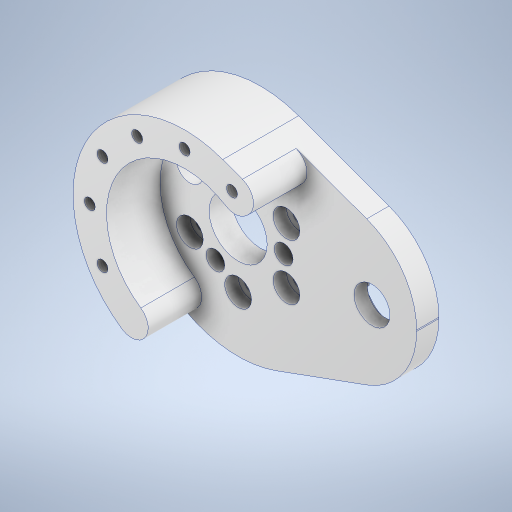
# Autodesk Inventor part: RP_Thigh-Base
Saved by Autodesk Inventor 2024.3 (Build 283343000, 343)
## iProperties
Created: 2024-10-20
Part Number: RP_Thigh-Base
Material: アルミニウム 6061
Document SubType Name: Sheet Metal
Designer: 佐藤智貴
Density: 2.7 g/cm^3
Appearance: アルミニウム - フラット
Mass: 44.9931 g
Surface Area: 86.4883 cm^2
Volume: 16.6641 cm^3
Sheet Metal Rule: Default
Author: 佐藤智貴
Autodesk Inventor part; units mm, degrees
ref_plane "YZ Plane" through (0, 0, 0) normal (1, 0, 0) x (0, 1, 0)
ref_plane "XZ Plane" through (0, 0, 0) normal (0, 1, 0) x (-1, 0, 0)
ref_plane "作業平面1" through (0, 0, 14) normal (0, 0, 1) x (-0.9659258, -0.258819, 0)
sketch "スケッチ14" plane through (0, 0, 0) normal (0, 0, 1) x (1, 0, 0)
  circle A0 centre (0, 0) radius 25
  circle A1 centre (30, 0) radius 4.025
  line L0 (0, 25) -> (40, 25)
  line L1 (40, 25) -> (40, -25)
  line L2 (40, -25) -> (0, -25)
  line L3 (0, -25) -> (0, 25)
  line L4 (0, -25) -> (40, -10.4412)
  line L5 (0, 25) -> (40, 10.4412)
  line L6 (0.5157, 26.4168) -> (40.5157, 11.858)
  line L7 (0.5157, -26.4168) -> (40.5157, -11.858)
  circle A2 centre (0, 0) radius 6.5
  line L8 (40.5157, -11.858) -> (63.847, -3.366)
  line L9 (37.8689, 40.3876) -> (23.4147, 35.1267)
  line L10 (23.4147, 35.1267) -> (-16.5853, 20.5679)
  line L11 (-16.5853, 20.5679) -> (-32.0428, 14.9418)
  line L12 (-32.0428, 14.9418) -> (-14.9418, -32.0428)
  line L13 (-14.9418, -32.0428) -> (0.5157, -26.4168)
  line L14 (40, 12.0456) -> (47.7428, -9.2275)
  line L15 (40, 12.0456) -> (30.6418, 37.7571)
  point P0 (8.5505, -23.4923)
  point P1 (40, -12.0456)
  point P2 (40, 12.0456)
  point P3 (8.5505, 23.4923)
  dimension "d111" = 50
  dimension "d112" = 8.05
  dimension "d113" = 30
  dimension "d114" = 40
  dimension "d115" = 50
  dimension "d116" = 25
  dimension "d119" = 25
  dimension "d126" = 20
  dimension "d127" = 20
  dimension "d144" = 13
  dimension "d201" = 90
  dimension "d202" = 90
  constraints: 32 end point, 5 collinear, 5 point on line, 4 parallel, 2 centre point, 2 coincident, 2 perpendicular, 1 horizontal, 1 midpoint, 8 other
  measures "d112" diameter of A1
  measures "d113" distance of point (0, 0) A1.centre
  measures "d114" distance of L0.start L0.end
  measures "d115" distance between parallel lines of L2 L0
  measures "d116" distance from line of point (0, 0) L0
  measures "d119" distance from line of L0 A1.centre
  measures "d126" angle of L0 L5
  measures "d127" angle of L2 L4
  measures "d144" diameter of A2
  measures "d201" angle of L13 L12
  measures "d202" angle of L8 L14
extrude "押し出し9" add sketch "スケッチ14" along normal blind 5 contours A0 L4 L3 A2 L5 | A0 L5 L1 L4 | L5 A0 | A0 L6 L1 L5 | L4 L1 L7 A0 | A0 L4 | L3 A2 A0
sketch "スケッチ15" plane through (0, 0, 0) normal (0, 0, -1) x (-1, 0, 0)
  circle A0 centre (-30, 0) radius 4.025 projected
  circle A1 centre (-30, 0) radius 6.6
  line L0 (-24.4, 3.4928) -> (-24.4, -3.4928)
  arc A2 (-24.4, 1.4928) -> (-24.4, 3.4928) centre (-24.4, 2.4928) ccw
  arc A3 (-24.4, -3.4928) -> (-24.4, -1.4928) centre (-24.4, -2.4928) ccw
  point P0 (0, 0)
  dimension "d122" = 13.2
  dimension "d203" = 5.6
  dimension "d204" = 1
  dimension "d205" = 1
  dimension "d206" = 0
  dimension "d207" = 0
  constraints: 6 point on circle, 3 centre point, 2 end point, 2 point on line, 1 coincident, 1 vertical
  measures "d122" diameter of A1
  measures "d203" distance from line of L0 A1.centre
  measures "d204" radius of A2
  measures "d205" radius of A3
  measures "d206" distance from line of L0 A2.centre
  measures "d207" distance from line of L0 A3.centre
extrude "押し出し10" cut sketch "スケッチ15" against normal blind 2 contours L0 A1 | A2 A1 | A1 A2 L0 | L0 A3 A1 | A1 A3
sketch "スケッチ16" plane through (0, 0, 5) normal (0, 0, 1) x (1, 0, 0)
  circle A0 centre (30, 0) radius 4.025 projected
  circle A1 centre (30, 0) radius 17
  arc A2 (8.5505, 23.4923) -> (8.5505, -23.4923) centre (0, 0) ccw projected
  circle A3 centre (0, 0) radius 25
  line L0 (40, -12.0456) -> (40, 12.0456) projected
  line L1 (40, 12.0456) -> (-0.2187, 26.6841)
  line L2 (40, -12.0456) -> (-2.6962, -27.5858)
  circle A4 centre (0, 0) radius 17.5
  line L3 (8.5505, 23.4923) -> (5.9854, 16.4446)
  line L4 (-17.5, 0) -> (-25, 0)
  line L5 (-2.7839, 19.6364) -> (32.5, 6.7941)
  line L6 (32.5, 6.7941) -> (32.5, -6.7941)
  line L7 (32.5, -6.7941) -> (-5.2613, -20.5381)
  line L8 (17.9474, 20.0721) -> (15.3823, 13.0244)
  line L9 (-17.5, 0) -> (0, 0)
  line L10 (-13.6656, -12.9367) -> (-0.4151, -19.1155)
  line L11 (-7.0404, -16.0261) -> (-11.4484, -25.4792)
  line L12 (17.2336, 18.1109) -> (11.4362, 13.2463)
  line L13 (18.0185, 5.7516) -> (7.3857, 18.4233)
  line L14 (0, 25) -> (0, 10.5586)
  line L15 (17.2336, 18.1109) -> (19.0798, 19.66)
  point P0 (0, -25)
  point P1 (-11.8057, -12.918)
  point P2 (-10.2087, -22.8207)
  point P3 (-7.3958, -15.8604)
  dimension "d125" = 34
  dimension "d128" = 7.5
  dimension "d164" = 7.5
  dimension "d165" = 10
  dimension "d186" = 90
  dimension "d187" = 65
  dimension "d196" = 30
  constraints: 30 end point, 8 point on circle, 4 tangent, 3 centre point, 3 coincident, 3 point on line, 2 perpendicular, 1 horizontal, 1 midpoint, 1 parallel, 1 vertical, 2 other
  measures "d125" diameter of A1
  measures "d128" radial gap between concentric circles of A3 A4
  measures "d164" distance between parallel lines of L1 L5
  measures "d165" distance between parallel lines of L8 L3
  measures "d186" angle of L10 L11
  measures "d187" angle of L4 L11
  measures "d196" angle of L3 L12
extrude "押し出し11" add sketch "スケッチ16" along normal blind 12 contours L12 L5 L3 A3 | A3 L1 L8 | L8 L1 L15 | L3 L5 L14 A2 | L12 L13 L5 | A2 L4 A4 L10 L11 | L14 A4 L4 A2 | L5 L13 L12 A4 | A4 L14 L5
sketch "スケッチ17" plane through (0, 0, 5) normal (0, 0, 1) x (1, 0, 0)
  circle A0 centre (30, 0) radius 4.025 projected
  line L0 (0, 0) -> (30, 0)
  circle A1 centre (0, 0) radius 12.5
  line L1 (0, 0) -> (12.4415, 7.1831)
  point P0 (10.8253, 6.25)
  point P1 (0, 12.5)
  point P2 (-10.8253, 6.25)
  point P3 (-10.8253, -6.25)
  point P4 (0, -12.5)
  point P5 (10.8253, -6.25)
  dimension "d131" = 25
  dimension "d132" = 30
  dimension "d135" = 360
  constraints: 4 end point, 1 coincident, 1 horizontal, 1 point on line, 10 other
  measures "d132" angle of L0 L1
hole "穴5" at (10.8253, 6.25, 5) at (0, 12.5, 5) at (-10.8253, 6.25, 5) at (-10.8253, -6.25, 5) at (0, -12.5, 5) at (10.8253, -6.25, 5) direction (0, 0, -1) diameter 3.2 end through all
sketch "スケッチ18" plane through (0, 0, 5) normal (0, 0, 1) x (1, 0, 0)
  circle A0 centre (30, 0) radius 4.025 projected
  line L0 (0, 0) -> (30, 0)
  circle A1 centre (0, 0) radius 10.2
  point P0 (10.2, 0)
  point P1 (-5.1, 8.8335)
  point P2 (-5.1, -8.8335)
  dimension "d145" = 20.4
  dimension "d148" = 360
  constraints: 2 end point, 1 coincident, 1 horizontal, 1 horizontal alignment, 1 point on line, 6 other
hole "穴6" at (10.2, 0, 5) at (-5.1, 8.8335, 5) at (-5.1, -8.8335, 5) direction (0, 0, -1) diameter 4.2 end through all
sketch "スケッチ19" plane through (0, 0, 5) normal (0, 0, 1) x (1, 0, 0)
  circle A0 centre (0, 12.5) radius 1.6 projected
  circle A1 centre (0, 0) radius 12.5
  circle A2 centre (0, 12.5) radius 3
  circle A3 centre (-10.8253, 6.25) radius 3
  circle A4 centre (-10.8253, -6.25) radius 3
  circle A5 centre (0, -12.5) radius 3
  circle A6 centre (10.8253, -6.25) radius 3
  circle A7 centre (10.8253, 6.25) radius 3
  dimension "d157" = 6
  dimension "d160" = 360
  constraints: 6 centre point, 2 coincident, 1 vertical alignment, 15 other
  measures "d157" diameter of A2
extrude "押し出し12" cut sketch "スケッチ19" against normal blind 3 contours A0 A1 | A0 A1 A2 | A1 A0 | A0 A1 A2 | A3 A1 | A1 A3 | A7 A1 | A1 A7 | A4 A1 | A1 A4 | A6 A1 | A1 A6 | A5 A1 | A1 A5
sketch "スケッチ20" plane through (0, 0, 17) normal (0, 0, 1) x (1, 0, 0)
  line L0 (19.0798, 19.66) -> (8.5505, 23.4923) projected
  line L1 (17.9474, 20.0721) -> (15.3823, 13.0244)
  line L2 (15.3823, 13.0244) -> (5.9854, 16.4446)
  line L3 (5.9854, 16.4446) -> (8.5505, 23.4923)
  line L4 (0, 0) -> (0, 30.7788)
  circle A0 centre (0, 0) radius 21.25
  circle A1 centre (0, 0) radius 25
  point P0 (11.9664, 18.2584)
  point P1 (0, 21.25)
  point P2 (-10.625, 18.403)
  point P3 (-18.403, 10.625)
  point P4 (-21.25, 0)
  point P5 (-18.403, -10.625)
  point P6 (-10.625, -18.403)
  point P7 (0, -21.25)
  point P8 (10.625, -18.403)
  point P9 (18.403, -10.625)
  point P10 (21.25, 0)
  point P11 (18.403, 10.625)
  point P12 (10.625, 18.403)
  dimension "d167" = 7.5
  dimension "d168" = 5
  dimension "d169" = 3.75
  dimension "d170" = 3.75
  dimension "d171" = 50
  dimension "d174" = 360
  constraints: 8 end point, 3 perpendicular, 2 coincident, 1 centre point, 1 point on line, 1 vertical, 1 vertical alignment, 15 other
  measures "d167" distance between parallel lines of L0 L2
  measures "d168" distance from line of L1 point (11.966, 18.258)
  measures "d169" distance from line of L2 point (11.966, 18.258)
  measures "d171" diameter of A1
hole "穴7" at (10.625, 18.403, 17) at (0, 21.25, 17) at (-10.625, 18.403, 17) at (-18.403, 10.625, 17) direction (0, 0, -1) diameter 2.459 depth 10 thread size "M3x0.5" class "6H" standard "ISO Metric profile"
fillet "フィレット9" radius 17 2 edges at (40, 12.0456, 2.5) (40, -12.0456, 2.5)
sketch "スケッチ21" plane through (0, 0, 17) normal (0, 0, 1) x (1, 0, 0)
  circle A0 centre (-18.403, 10.625) radius 1.2295 projected
  circle A1 centre (0, 0) radius 21.25
  line L0 (0, 0) -> (-31.1052, 0)
  point P0 (-21.25, 0)
  point P1 (-18.403, -10.625)
  constraints: 2 coincident, 2 end point, 2 point on circle, 1 centre point, 1 horizontal, 1 symmetric about line
hole "穴8" at (-21.25, 0, 17) at (-18.403, -10.625, 17) direction (0, 0, -1) diameter 2.459 depth 10 thread size "M3x0.5" class "6H" standard "ISO Metric profile"
fillet "フィレット12" radius 3.75 4 edges at (-7.0404, -16.0261, 11) (-10.2087, -22.8207, 11) (19.0798, 19.66, 11) (11.4362, 13.2463, 11)
